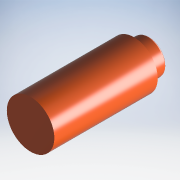
# Autodesk Inventor part: Pok X-Carriage Bottom Support
Saved by Autodesk Inventor 2018.2 (Build 222227000, 227)
## iProperties
Created: 2018-02-07
Part Number: Pok X-Carriage Bottom Support
Material: ABS Plastic
Document SubType Name: Modeling
Designer: Moochster
Density: 1.06 g/cm^3
Appearance: Smooth - Light Orange
Author: Moochster
Autodesk Inventor part; units mm, degrees
ref_plane "YZ Plane" through (0, 0, 0) normal (1, 0, 0) x (0, 1, 0)
ref_plane "XZ Plane" through (0, 0, 0) normal (0, 1, 0) x (-1, 0, 0)
ref_plane "XY Plane" through (0, 0, 0) normal (0, 0, 1) x (1, 0, 0)
sketch "Sketch1" plane through (0, 0, 0) normal (0, 0, 1) x (1, 0, 0)
  line L0 (0, 0) -> (0, 20)
  line L1 (2.85, 20) -> (2.85, 17.4)
  line L2 (2.85, 17.4) -> (4, 17.4)
  line L3 (4, 17.4) -> (4, 0)
  line L4 (4, 0) -> (0, 0)
  line L5 (2.85, 20) -> (1.65, 20)
  line L6 (1.65, 20) -> (1.65, 12)
  line L7 (1.65, 12) -> (0, 12)
  dimension "d0" = 8
  dimension "d1" = 5.7
  dimension "d2" = 2.6
  dimension "d3" = 20
  dimension "d6" = 3.3
  dimension "d7" = 8
  constraints: 16 end point, 4 perpendicular, 2 horizontal, 1 horizontal alignment, 1 point on line, 1 vertical
  measures "d0" diameter of L3 L0
  measures "d1" diameter of L1 L0
  measures "d2" distance of L1.start L1.end
  measures "d3" distance of L0.start L0.end
  measures "d6" diameter of L6 L0
  measures "d7" distance of L5.end L6.end
revolve "Revolution1" add sketch "Sketch1" angle 360 about axis through (0, 0, 0) along (0, 1, 0)
fillet "Fillet1" radius 0.3 1 edges at (-2.85, 20, 0)
body "Solid1"
